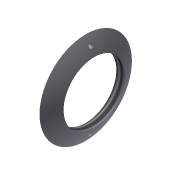
# Autodesk Inventor part: retainingring
Saved by Autodesk Inventor 2015 (Build 190159000, 159)
## iProperties
Created: 2015-10-30
Part Number: retainingring
Material: Generic
Document SubType Name: Modeling
Designer: jad211
Density: 1 g/cm^3
Appearance: Default
Author: jad211
Autodesk Inventor part; units mm, degrees
ref_plane "YZ Plane" through (0, 0, 0) normal (1, 0, 0) x (0, 1, 0)
ref_plane "XZ Plane" through (0, 0, 0) normal (0, 1, 0) x (-1, 0, 0)
ref_plane "XY Plane" through (0, 0, 0) normal (0, 0, 1) x (1, 0, 0)
sketch "Sketch1" plane through (0, 0, 0) normal (0, 1, 0) x (-1, 0, 0)
  arc A0 (-71.9659, -29.6) -> (-63.7659, -44.6) centre (0, 0) ccw
  line L0 (-63.7659, -29.6) -> (-71.9659, -29.6)
  line L1 (-63.7659, -29.6) -> (-63.7659, -44.6)
  line L2 (14.4758, 0) -> (-86.8548, 0) projected
  dimension "d1" = 15
  dimension "d2" = 8.2
  dimension "d4" = 29.6
  constraints: 4 end point, 2 point on circle, 1 centre point, 1 coincident, 1 horizontal, 1 perpendicular
  measures "d1" distance of L0.start L1.end
  measures "d2" distance of L0.start L0.end
  measures "d4" distance from line of point (0, 0) L0
revolve "Revolution1" add sketch "Sketch1" angle 360 about axis through (-10, 0, 0) along (1, 0, 0)
thread "Thread1" size "M60x5.5" class "6H" standard "ANSI Metric M Profile" full length
sketch "Sketch2" plane through (63.7659, 0, 0) normal (-1, 0, 0) x (0, 0, 1)
  circle A0 centre (-37, 0) radius 1.75
  circle A1 centre (37, 0) radius 1.75
  point P0 (0, 0)
  dimension "d8" = 74
  dimension "d9" = 37
  dimension "d12" = 3.5
  dimension "d13" = 3.5
  constraints: 2 centre point
  measures "d8" distance of A1.centre A0.centre
  measures "d9" distance of point (0, 0) A1.centre
  measures "d12" diameter of A0
  measures "d13" diameter of A1
extrude "Extrusion1" cut sketch "Sketch2" against normal up to next
equation "\"d9\" = 0.5 * d8"
body "Solid1"
